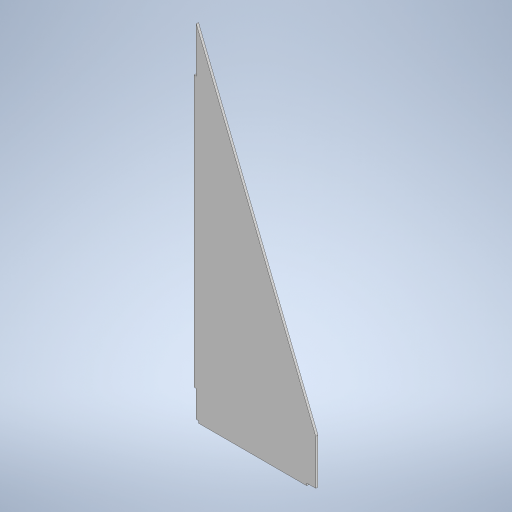
# Autodesk Inventor part: side support
Saved by Autodesk Inventor 2023 (Build 270158000, 158)
## iProperties
Created: 2023-10-15
Part Number: side support
Material: Generic
Document SubType Name: Modeling
Designer: Nate
Density: 1 g/cm^3
Appearance: Default
Author: Nate
Autodesk Inventor part; units mm, degrees
ref_plane "YZ Plane" through (0, 0, 0) normal (1, 0, 0) x (0, 1, 0)
ref_plane "XZ Plane" through (0, 0, 0) normal (0, 1, 0) x (-1, 0, 0)
ref_plane "XY Plane" through (0, 0, 0) normal (0, 0, 1) x (1, 0, 0)
sketch "Sketch1" plane through (0, 0, 0) normal (0, 0, 1) x (1, 0, 0)
  line L0 (0, 0) -> (152.4, 0)
  line L1 (152.4, 0) -> (152.4, 3.175)
  line L2 (152.4, 3.175) -> (0, 3.175)
  line L3 (0, 3.175) -> (0, 0)
  line L4 (0, 3.175) -> (11.1125, 3.175)
  line L5 (152.4, 3.175) -> (190.5, 3.175)
  line L6 (0, 3.175) -> (11.1125, 3.175)
  line L7 (0, 3.175) -> (-3.175, 3.175)
  line L8 (-3.175, 3.175) -> (-3.175, 485.775)
  line L9 (-3.175, 485.775) -> (0, 485.775)
  line L10 (0, 485.775) -> (0, 3.175)
  line L11 (-3.175, 40.7756) -> (-6.35, 40.7756)
  line L12 (-6.35, 40.7756) -> (-6.35, 421.7756)
  line L13 (-6.35, 421.7756) -> (-3.175, 421.7756)
  line L14 (-3.175, 421.7756) -> (-3.175, 40.7756)
  line L15 (190.5, 3.175) -> (-3.175, 485.775)
  line L16 (165.1, 3.175) -> (165.1, 66.675)
  line L17 (165.1, 3.175) -> (228.6, 3.175) construction
  point P0 (5.5563, 3.175)
  point P1 (-1.5875, 3.175)
  point P2 (-4.7625, 40.7756)
  point P3 (-3.175, 421.7756)
  point P4 (165.1, 66.4668)
  dimension "d0" = 152.4
  dimension "d1" = 3.175
  dimension "d7" = 38.1
  dimension "d15" = 3.175
  dimension "d16" = 482.6
  dimension "d17" = 3.175
  dimension "d18" = 381
  dimension "d19" = 37.6006
  dimension "d20" = 63.5
  dimension "d21" = 90
  dimension "d22" = 25.4
  constraints: 36 end point, 7 horizontal, 6 parallel, 4 perpendicular, 3 midpoint, 2 point on line, 1 vertical
  measures "d0" distance of L2.end L1.end
  measures "d1" distance of L1.end L0.end
  measures "d7" distance of L1.end L5.end
  measures "d15" distance between parallel lines of L10 L8
  measures "d16" distance from line of point (-1.588, 3.175) L9
  measures "d17" distance of L12.end L13.end
  measures "d18" distance of L11.end L12.end
  measures "d19" distance from line of L2 point (-4.763, 40.776)
  measures "d20" distance of L16.start L16.end
  measures "d21" angle of L17 L16
  measures "d22" distance from line of L5.end L16
extrude "Extrusion1" add sketch "Sketch1" along normal blind 3.175 contours L3 L2 L1 L0 | L10 L15 L16 L5 L2 | L7 L8 L15 L10 | L11 L12 L13 L8
body "Solid1"
